Autodesk Inventor part; units mm, degrees
(part 2 of 2)
sketch "Sketch6" plane through (0, 0, 0) normal (0, 0, -1) x (-1, 0, 0)
  circle A0 centre (-10.8188, 61.3387) radius 1.5 projected
  circle A1 centre (-68.6105, -28.321) radius 1.63 projected
  arc A2 (-88.5111, 275.0837) -> (-92.5111, 275.0837) centre (-90.5111, 275.0837) ccw projected
  line L0 (-88.5111, 275.0837) -> (-88.5111, 230.0837) projected
  arc A3 (-92.5111, 230.0837) -> (-88.5111, 230.0837) centre (-90.5111, 230.0837) ccw projected
  line L1 (-92.5111, 230.0837) -> (-92.5111, 275.0837) projected
  arc A4 (-43.5111, 275.0837) -> (-47.5111, 275.0837) centre (-45.5111, 275.0837) ccw projected
  line L2 (-43.5111, 275.0837) -> (-43.5111, 230.0837) projected
  arc A5 (-47.5111, 230.0837) -> (-43.5111, 230.0837) centre (-45.5111, 230.0837) ccw projected
  line L3 (-47.5111, 230.0837) -> (-47.5111, 275.0837) projected
  circle A6 centre (-6.132, -79.3472) radius 1.25 projected
  circle A7 centre (-145.3842, 185.8247) radius 1.5 projected
  circle A8 centre (-153.8932, -1.3222) radius 1.5 projected
  circle A9 centre (-145.3842, -79.3472) radius 1.5 projected
  circle A10 centre (-129.8902, 6.8528) radius 1.5 projected
  circle A11 centre (-116.3012, -71.1722) radius 1.5 projected
  circle A12 centre (-129.8902, 272.0247) radius 1.5 projected
  circle A13 centre (-129.8902, 185.8247) radius 1.5 projected
  circle A14 centre (-116.3012, 263.8497) radius 1.5 projected
  circle A15 centre (17.871, -71.1722) radius 1.5 projected
  circle A16 centre (-6.132, 6.8528) radius 1.5 projected
  circle A17 centre (-19.721, -1.3222) radius 1.5 projected
  circle A18 centre (17.871, 263.8497) radius 1.5 projected
  circle A19 centre (9.362, 272.0247) radius 1.5 projected
  circle A20 centre (9.362, 185.8247) radius 1.5 projected
  circle A21 centre (-19.721, 193.9997) radius 1.5 projected
  circle A22 centre (-19.721, 263.8497) radius 1.5 projected
  circle A23 centre (-6.132, 185.8247) radius 1.5 projected
  circle A24 centre (-6.132, 272.0247) radius 1.5 projected
  circle A25 centre (17.871, 193.9997) radius 1.5 projected
  circle A26 centre (-19.721, -71.1722) radius 1.5 projected
  circle A27 centre (9.362, -79.3472) radius 1.5 projected
  circle A28 centre (9.362, 6.8528) radius 1.5 projected
  circle A29 centre (17.871, -1.3222) radius 1.5 projected
  circle A30 centre (-116.3012, 193.9997) radius 1.5 projected
  circle A31 centre (-153.8932, 193.9997) radius 1.5 projected
  circle A32 centre (-153.8932, 263.8497) radius 1.5 projected
  circle A33 centre (-145.3842, 6.8528) radius 1.5 projected
  circle A34 centre (-129.8902, -79.3472) radius 1.5 projected
  circle A35 centre (-153.8932, -71.1722) radius 1.5 projected
  circle A36 centre (-116.3012, -1.3222) radius 1.5 projected
  circle A37 centre (-145.3842, 272.0247) radius 1.5 projected
  arc A38 (81.2372, 206.8201) -> (56.4499, 266.1206) centre (-44.5185, 189.0856) ccw projected
  ellipse E0 centre (-68.0111, 96.3387) end of major axis (-68.0111, -141.4053) minor radius 177.8 (56.4499, 266.1206) -> (-192.4721, 266.1206) ccw projected
  arc A39 (-192.4721, 266.1206) -> (-217.2594, 206.8201) centre (-91.5037, 189.0856) ccw projected
  arc A40 (-217.2594, 206.8201) -> (-217.2594, -14.1426) centre (566.1677, 96.3387) ccw projected
  arc A41 (-217.2594, -14.1426) -> (-192.4721, -73.4431) centre (-91.5037, 3.5918) ccw projected
  ellipse E1 centre (-68.0111, 96.3387) end of major axis (-68.0111, -141.4053) minor radius 177.8 (-192.4721, -73.4431) -> (56.4499, -73.4431) ccw projected
  arc A42 (56.4499, -73.4431) -> (81.2372, -14.1426) centre (-44.5185, 3.5918) ccw projected
  arc A43 (81.2372, -14.1426) -> (81.2372, 206.8201) centre (-702.1899, 96.3387) ccw projected
  circle A44 centre (-35.6216, 248.9087) radius 1.25 projected
  circle A45 centre (-100.4006, 318.7587) radius 1.25 projected
  circle A46 centre (-100.4006, 248.9087) radius 1.25 projected
  circle A47 centre (-35.6216, 318.7587) radius 1.25 projected
  circle A48 centre (-56.9111, -118.4053) radius 1.5 projected
  circle A49 centre (-79.1111, -118.4053) radius 1.5 projected
  circle A50 centre (-58.7361, -128.5803) radius 1.5 projected
  circle A51 centre (-61.0891, -46.904) radius 1.5 projected
  circle A52 centre (-53.9141, -54.079) radius 1.5 projected
  circle A53 centre (-92.2681, -54.079) radius 1.5 projected
  circle A54 centre (-85.0931, -46.904) radius 1.5 projected
  circle A55 centre (-77.2861, -128.5803) radius 1.5 projected
  circle A56 centre (-79.1111, -110.4053) radius 1.5 projected
  circle A57 centre (-56.9111, -110.4053) radius 1.5 projected
  line L4 (-82.971, -17.5241) -> (-82.971, 43.3967) projected
  line L5 (-82.971, 43.3967) -> (-52.491, 43.3967) projected
  line L6 (-52.491, 43.3967) -> (-52.491, -17.5241) projected
  line L7 (-52.491, -17.5241) -> (-82.971, -17.5241) projected
  circle A58 centre (-68.0111, 137.616) radius 35 projected
  line L8 (-123.7158, 171.3631) -> (-119.7158, 171.3631) projected
  arc A59 (-119.7158, 168.3632) -> (-119.7158, 171.3631) centre (-119.7158, 169.8631) ccw projected
  line L9 (-119.7158, 168.3632) -> (-123.7158, 168.3632) projected
  arc A60 (-123.7158, 171.3631) -> (-123.7158, 168.3632) centre (-123.7158, 169.8631) ccw projected
  line L10 (-123.6698, 106.6744) -> (-119.6698, 106.6744) projected
  arc A61 (-119.6698, 103.6746) -> (-119.6698, 106.6744) centre (-119.6698, 105.1745) ccw projected
  line L11 (-119.6698, 103.6746) -> (-123.6698, 103.6746) projected
  arc A62 (-123.6698, 106.6744) -> (-123.6698, 103.6746) centre (-123.6698, 105.1745) ccw projected
  line L12 (-9.1669, 171.4444) -> (-5.1669, 171.4444) projected
  arc A63 (-5.1669, 168.4446) -> (-5.1669, 171.4444) centre (-5.1669, 169.9445) ccw projected
  line L13 (-5.1669, 168.4446) -> (-9.1669, 168.4446) projected
  arc A64 (-9.1669, 171.4444) -> (-9.1669, 168.4446) centre (-9.1669, 169.9445) ccw projected
  line L14 (-5.1669, 103.6742) -> (-9.1669, 103.6742) projected
  arc A65 (-9.1669, 106.6741) -> (-9.1669, 103.6742) centre (-9.1669, 105.1742) ccw projected
  line L15 (-9.1669, 106.6741) -> (-5.1669, 106.6741) projected
  arc A66 (-5.1669, 103.6742) -> (-5.1669, 106.6741) centre (-5.1669, 105.1742) ccw projected
  arc A67 (-34.0816, 86.6493) -> (-37.0792, 86.6494) centre (-35.5804, 86.6492) ccw projected
  line L16 (-34.0816, 86.6493) -> (-34.0814, 82.6493) projected
  arc A68 (-37.0794, 82.6493) -> (-34.0814, 82.6493) centre (-35.5804, 82.6492) ccw projected
  line L17 (-37.0794, 82.6493) -> (-37.0792, 86.6494) projected
  arc A69 (-34.0865, 201.0395) -> (-37.0841, 201.0395) centre (-35.5853, 201.0395) ccw projected
  line L18 (-34.0865, 201.0395) -> (-34.0863, 197.0396) projected
  arc A70 (-37.0843, 197.0395) -> (-34.0863, 197.0396) centre (-35.5853, 197.0395) ccw projected
  line L19 (-37.0843, 197.0395) -> (-37.0841, 201.0395) projected
  arc A71 (-34.0812, 78.9993) -> (-37.0788, 78.9992) centre (-35.58, 78.9992) ccw projected
  line L20 (-34.0812, 78.9993) -> (-34.081, 74.9993) projected
  arc A72 (-37.079, 74.9993) -> (-34.081, 74.9993) centre (-35.58, 74.9992) ccw projected
  line L21 (-37.079, 74.9993) -> (-37.0788, 78.9992) projected
  arc A73 (-98.9325, 193.3865) -> (-101.9301, 193.3866) centre (-100.4313, 193.3865) ccw projected
  line L22 (-98.9325, 193.3865) -> (-98.9323, 189.3866) projected
  arc A74 (-101.9303, 189.3866) -> (-98.9323, 189.3866) centre (-100.4313, 189.3865) ccw projected
  line L23 (-101.9303, 189.3866) -> (-101.9301, 193.3866) projected
  circle A75 centre (-95.163, -4.4165) radius 1.25 projected
  circle A76 centre (-36.616, 37.0467) radius 1.25 projected
  circle A77 centre (-46.141, -14.3491) radius 1.25 projected
  circle A78 centre (-36.616, -11.1741) radius 1.25 projected
  circle A79 centre (-36.616, 12.9421) radius 1.25 projected
  circle A80 centre (-46.141, 40.2217) radius 1.25 projected
  circle A81 centre (-95.163, 40.4375) radius 1.25 projected
  arc A82 (-98.8512, 78.9533) -> (-101.8488, 78.9533) centre (-100.35, 78.9533) ccw projected
  line L24 (-98.8512, 78.9533) -> (-98.851, 74.9533) projected
  arc A83 (-101.849, 74.9533) -> (-98.851, 74.9533) centre (-100.35, 74.9533) ccw projected
  line L25 (-101.849, 74.9533) -> (-101.8488, 78.9533) projected
  line L26 (-34.0865, 193.3895) -> (-34.0863, 189.3896) projected
  arc A84 (-37.0843, 189.3896) -> (-34.0863, 189.3896) centre (-35.5853, 189.3895) ccw projected
  line L27 (-37.0843, 189.3896) -> (-37.0841, 193.3896) projected
  arc A85 (-34.0865, 193.3895) -> (-37.0841, 193.3896) centre (-35.5853, 193.3895) ccw projected
  arc A86 (-98.9379, 201.0395) -> (-101.9362, 200.9947) centre (-100.4367, 200.9934) ccw projected
  line L28 (-98.9379, 201.0395) -> (-98.9377, 196.9935) projected
  arc A87 (-101.9357, 196.9932) -> (-98.9377, 196.9935) centre (-100.4367, 196.9934) ccw projected
  line L29 (-101.9357, 196.9932) -> (-101.9362, 200.9947) projected
  arc A88 (-98.8567, 86.6032) -> (-101.8543, 86.6033) centre (-100.3555, 86.6032) ccw projected
  line L30 (-98.8567, 86.6032) -> (-98.8565, 82.6033) projected
  arc A89 (-101.8544, 82.6033) -> (-98.8565, 82.6033) centre (-100.3555, 82.6032) ccw projected
  line L31 (-101.8544, 82.6033) -> (-101.8543, 86.6033) projected
  line L32 (-16.8169, 106.6744) -> (-12.8169, 106.6744) projected
  arc A90 (-12.8169, 103.6746) -> (-12.8169, 106.6744) centre (-12.8169, 105.1745) ccw projected
  line L33 (-12.8169, 103.6746) -> (-16.8169, 103.6746) projected
  arc A91 (-16.8169, 106.6744) -> (-16.8169, 103.6746) centre (-16.8169, 105.1745) ccw projected
  line L34 (-16.8629, 171.439) -> (-12.8629, 171.439) projected
  arc A92 (-12.8629, 168.4391) -> (-12.8629, 171.439) centre (-12.8629, 169.9391) ccw projected
  line L35 (-12.8629, 168.4391) -> (-16.8629, 168.4391) projected
  arc A93 (-16.8629, 171.439) -> (-16.8629, 168.4391) centre (-16.8629, 169.9391) ccw projected
  line L36 (-131.3198, 106.6744) -> (-127.3198, 106.6744) projected
  arc A94 (-127.3198, 103.6746) -> (-127.3198, 106.6744) centre (-127.3198, 105.1745) ccw projected
  line L37 (-127.3198, 103.6746) -> (-131.3198, 103.6746) projected
  arc A95 (-131.3198, 106.6744) -> (-131.3198, 103.6746) centre (-131.3198, 105.1745) ccw projected
  line L38 (-131.3658, 171.3576) -> (-127.3658, 171.3576) projected
  arc A96 (-127.3658, 168.3578) -> (-127.3658, 171.3576) centre (-127.3658, 169.8577) ccw projected
  line L39 (-127.3658, 168.3578) -> (-131.3658, 168.3578) projected
  arc A97 (-131.3658, 171.3576) -> (-131.3658, 168.3578) centre (-131.3658, 169.8577) ccw projected
  circle A98 centre (-10.8188, 71.3387) radius 1.5 projected
  line L40 (-5.9653, 56.3387) -> (-15.6724, 56.3387) projected
  line L41 (-3.9653, 100.9185) -> (-3.9653, 58.3387) projected
  arc A99 (-5.9653, 56.3387) -> (-3.9653, 58.3387) centre (-5.9653, 58.3387) ccw projected
  arc A100 (-17.6724, 58.3387) -> (-15.6724, 56.3387) centre (-15.6724, 58.3387) ccw projected
  line L42 (-17.6724, 58.3387) -> (-17.6724, 100.9185) projected
  line L43 (-16.6724, 101.9185) -> (-4.9653, 101.9185) projected
  arc A101 (-3.9653, 100.9185) -> (-4.9653, 101.9185) centre (-4.9653, 100.9185) ccw projected
  arc A102 (-16.6724, 101.9185) -> (-17.6724, 100.9185) centre (-16.6724, 100.9185) ccw projected
  line L44 (-3.9653, 100.9185) -> (-3.9653, 58.3387) projected
  line L45 (-3.9653, 100.9185) -> (-3.9653, 58.3387)
  line L46 (-3.9653, 114.3387) -> (-3.9653, 78.3387) projected
  line L47 (-3.9653, 101.4185) -> (-3.9653, 79.6285)
  line L48 (-3.9653, 79.6285) -> (-17.6724, 79.6286)
  circle A103 centre (-125.2036, 96.9184) radius 1.75 projected
  circle A104 centre (-10.8185, 96.9184) radius 1.75 projected
  circle A105 centre (-10.8187, 86.9184) radius 1.75 projected
  circle A106 centre (-125.2035, 86.9184) radius 1.75 projected
  circle A107 centre (-125.2039, 71.3387) radius 1.75 projected
  circle A108 centre (-10.8188, 71.3387) radius 1.75 projected
  circle A109 centre (-10.8188, 61.3387) radius 1.75 projected
  circle A110 centre (-125.2039, 61.3387) radius 1.75 projected
  circle A111 centre (-10.8187, 86.9184) radius 1.5
  circle A112 centre (-10.8185, 96.9184) radius 1.5
  point P0 (0, 0)
  dimension "d26" = 21.79
  dimension "d29" = 3
  dimension "d30" = 3
  constraints: 6 end point, 2 centre point, 2 coincident, 2 point on line, 1 collinear, 1 midpoint, 2 other
  measures "d26" distance of L47.start L47.end
  measures "d29" diameter of A111
  measures "d30" diameter of A112
extrude "Extrusion5" cut sketch "Sketch6" against normal blind 10 contours A111 | A112
body "Solid1"
